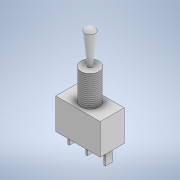
# Autodesk Inventor part: switch-mockup
Saved by Autodesk Inventor 2021 (Build 250183000, 183)
## iProperties
Created: 2024-04-22
Part Number: switch-mockup
Material: Generic
Document SubType Name: Modeling
Designer: Toby
Density: 1 g/cm^3
Appearance: Default
Author: Toby
Autodesk Inventor part; units mm, degrees
ref_plane "YZ Plane" through (0, 0, 0) normal (1, 0, 0) x (0, 1, 0)
ref_plane "XZ Plane" through (0, 0, 0) normal (0, 1, 0) x (-1, 0, 0)
ref_plane "XY Plane" through (0, 0, 0) normal (0, 0, 1) x (1, 0, 0)
sketch "Sketch1" plane through (0, 0, 0) normal (0, 0, 1) x (1, 0, 0)
  line L0 (-6.5, 4.5) -> (6.5, 4.5)
  line L1 (6.5, 4.5) -> (6.5, -4.5)
  line L2 (6.5, -4.5) -> (-6.5, -4.5)
  line L3 (-6.5, -4.5) -> (-6.5, 4.5)
  point P0 (0, 0)
  dimension "d0" = 13
  dimension "d1" = 9
  dimension "d2" = 4.5
  dimension "d3" = 6.5
  constraints: 8 end point, 2 parallel, 1 horizontal, 1 perpendicular
  measures "d0" distance of L0.start L0.end
  measures "d1" distance of L2.end L0.start
  measures "d2" distance from line of point (0, 0) L0
  measures "d3" distance from line of L3 point (0, 0)
extrude "Extrusion1" add sketch "Sketch1" along normal blind 7
sketch "Sketch2" plane through (-6.5, -4.5, 0) normal (0, -1, 0) x (1, 0, 0)
  line L0 (1, 4.5) -> (1.5, 4.5)
  line L1 (1.5, 4.5) -> (1.5, 2.5)
  line L2 (1.5, 2.5) -> (1, 2.5)
  line L3 (1, 2.5) -> (1, 4.5)
  line L4 (11.5, 4.5) -> (12, 4.5)
  line L5 (12, 4.5) -> (12, 2.5)
  line L6 (12, 2.5) -> (11.5, 2.5)
  line L7 (11.5, 2.5) -> (11.5, 4.5)
  line L8 (6.25, 2.5) -> (6.75, 2.5)
  line L9 (6.75, 2.5) -> (6.75, 4.5)
  line L10 (6.75, 4.5) -> (6.25, 4.5)
  line L11 (6.25, 4.5) -> (6.25, 2.5)
  line L12 (0, 0) -> (0, 7) projected
  line L13 (13, 0) -> (13, 7) projected
  line L14 (0, 7) -> (13, 7) projected
  point P0 (6.5, 0)
  dimension "d6" = 0.5
  dimension "d7" = 0.5
  dimension "d8" = 0.5
  dimension "d9" = 1
  dimension "d10" = 1
  dimension "d11" = 6.25
  dimension "d12" = 6.25
  dimension "d13" = 2
  dimension "d14" = 2
  dimension "d15" = 2
  dimension "d16" = 2.5
  constraints: 24 end point, 6 parallel, 3 horizontal, 3 perpendicular, 3 point on line
  measures "d6" distance between parallel lines of L1 L3
  measures "d7" distance between parallel lines of L11 L9
  measures "d8" distance between parallel lines of L5 L7
  measures "d9" distance between parallel lines of L12 L3
  measures "d10" distance between parallel lines of L13 L5
  measures "d11" distance between parallel lines of L13 L9
  measures "d12" distance between parallel lines of L12 L11
  measures "d13" distance between parallel lines of L2 L0
  measures "d14" distance between parallel lines of L8 L10
  measures "d15" distance between parallel lines of L6 L4
  measures "d16" distance between parallel lines of L0 L14
extrude "Extrusion2" add sketch "Sketch2" along normal blind 4
sketch "Sketch3" plane through (-6.5, 4.5, 0) normal (0, 1, 0) x (1, 0, 0)
  line L0 (0, -7) -> (13, -7) projected
  line L1 (0, 0) -> (0, -7) projected
  circle A0 centre (6.5, -3.5) radius 2.65
  point P0 (6.5, 0)
  point P1 (6.5, -7)
  point P2 (0, -3.5)
  dimension "d19" = 5.3
  constraints: 2 midpoint, 1 centre point, 1 coincident
  measures "d19" diameter of A0
extrude "Extrusion3" add sketch "Sketch3" along normal blind 9
sketch "Sketch4" plane through (0, 13.5, 3.5) normal (0, 1, 0) x (1, 0, 0)
  line L0 (-0.5, 0) -> (0.5, 0)
  line L1 (0.5, 0) -> (0.5, 0.1)
  line L2 (0.5, 0.1) -> (-0.5, 0.1)
  line L3 (-0.5, 0.1) -> (-0.5, 0)
  circle A0 centre (0, 0) radius 2.65 projected
  point P0 (0, 3.5)
  dimension "d22" = 0
  dimension "d23" = 0.1
  dimension "d24" = 0.5
  dimension "d25" = 0.5
  constraints: 8 end point, 2 parallel, 1 horizontal, 1 perpendicular
  measures "d22" distance from line of A0.centre L0
  measures "d23" distance between parallel lines of L0 L2
  measures "d24" distance from line of A0.centre L3
  measures "d25" distance from line of A0.centre L1
extrude "Extrusion4" add sketch "Sketch4" along normal blind 3 contours L3 L2 L1 L0
sketch "Sketch5" plane through (-0.5, 13.5, 3.5) normal (0, 0, 1) x (1, 0, 0)
  line L0 (3.15, 0) -> (-2.15, 0) projected
  line L1 (0, 0) -> (0, 3) projected
  line L2 (1.1, 0) -> (2, 9)
  arc A0 (2, 9) -> (0.5, 10) centre (0.5167, 8.4001) ccw
  line L3 (0.5, 10) -> (0.5, 0)
  line L4 (1.1, 0) -> (0.5, 0)
  line L5 (0.5, -28.4463) -> (0.5, 16.6776) projected
  point P0 (0.5, -13.5)
  point P1 (2, 10)
  dimension "d28" = 10
  dimension "d29" = 1.5
  dimension "d30" = 1.1
  dimension "d31" = 1
  dimension "d32" = 1.6
  constraints: 6 end point, 2 point on circle, 1 centre point, 1 midpoint, 1 perpendicular, 1 point on line, 1 vertical
  measures "d28" distance from line of L0 L3.start
  measures "d29" distance of L3.start point (2, 10)
  measures "d30" distance from line of L1 L2.start
  measures "d31" distance of L2.end point (2, 10)
  measures "d32" radius of A0
revolve "Revolution1" add sketch "Sketch5" angle 360 about axis through (0, -10, 3.5) along (0, 1, 0)
thread "Thread1" size "M5.5x0.5" class "6g" standard "ANSI Metric M Profile" full length
body "Solid1"
